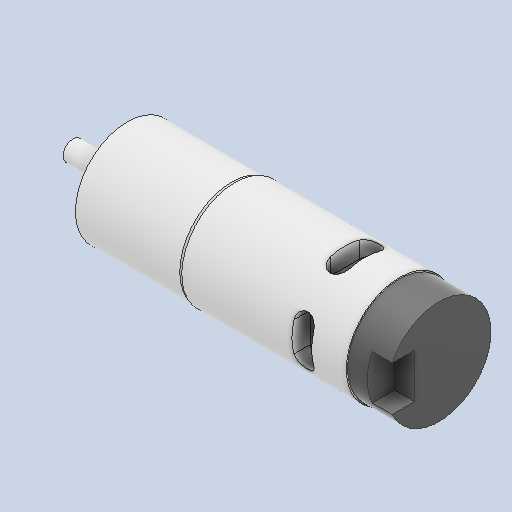
# Autodesk Inventor part: CHP-42GP-775 ABHL
Saved by Autodesk Inventor 2025 (Build 290162000, 162)
## iProperties
Created: 2025-02-16
Part Number: CHP-42GP-775 ABHL
Material: Типовые
Document SubType Name: Modeling
Designer: volko
Density: 1 g/cm^3
Appearance: По умолчанию
Finish1_Area: 8378,395 мм^2
Finish1_Appearance: Smooth - White
Finish2_Area: 1962,332 мм^2
Finish2_Appearance: Glossy - Black
Finish3_Area: 3635,353 мм^2
Finish3_Appearance: Smooth - Black
Finish4_Area: 9380,563 мм^2
Finish4_Appearance: Smooth - White
Author: volko
Autodesk Inventor part; units mm, degrees
ref_plane "YZ Plane" through (0, 0, 0) normal (1, 0, 0) x (0, 1, 0)
ref_plane "XZ Plane" through (0, 0, 0) normal (0, 1, 0) x (-1, 0, 0)
sketch "Эскиз1" plane through (0, 0, 0) normal (0, 0, 1) x (1, 0, 0)
  line L0 (0, 0) -> (0, 4)
  line L1 (0, 4) -> (20, 4)
  line L2 (20, 4) -> (20, 13)
  line L3 (20, 13) -> (22, 13)
  line L4 (22, 13) -> (22, 21)
  line L5 (22, 21) -> (65.5, 21)
  line L6 (65.5, 21.5) -> (132, 21.5)
  line L7 (132, 21.5) -> (132, 21)
  line L8 (132, 21) -> (148, 21)
  line L9 (148, 21) -> (148, 0)
  line L10 (0, 0) -> (148, 0)
  line L11 (65.5, 21) -> (65.5, 21.5)
  point P0 (63, 17.5)
  point P1 (63, 17.5)
  dimension "d5" = 22
  dimension "d6" = 2
  dimension "d7" = 8
  dimension "d8" = 26
  dimension "d9" = 42
  dimension "d11" = 43
  dimension "d12" = 43.5
  dimension "d14" = 66.5
  dimension "d15" = 16
  constraints: 24 end point, 7 perpendicular, 3 vertical, 1 coincident, 1 collinear, 1 parallel, 2 other
  measures "d5" distance between parallel lines of L0 L4
  measures "d6" distance between parallel lines of L2 L4
  measures "d7" diameter of L1 L10
  measures "d8" diameter of L3 L10
  measures "d9" diameter of L5 L10
  measures "d11" diameter of L6 L10
  measures "d12" distance of L4.end L5.end
  measures "d14" distance between parallel lines of L7 L11
  measures "d15" distance of L7.end L8.end
revolve "Вращение1" add sketch "Эскиз1" angle 360 about axis through (0, 0, 0) along (1, 0, 0)
fillet "Сопряжение1" radius 2 1 edges at (65.5, -21, 0)
sketch "Эскиз2" plane through (0, 0, 0) normal (0, 1, 0) x (-1, 0, 0)
  line L0 (0, 4) -> (0, -4) projected
  line L1 (0, -3.5) -> (-12, -3.5)
  line L2 (-12, -3.5) -> (-12, -6.5419)
  line L3 (-12, -6.5419) -> (0, -6.5419)
  line L4 (0, -3.1455) -> (0, -6.5419)
  point P0 (0, 0)
  point P1 (0, 0)
  dimension "d20" = 3.5
  dimension "d21" = 12
  constraints: 8 end point, 2 perpendicular, 2 point on line, 1 horizontal, 1 midpoint, 1 vertical
  measures "d20" distance from line of point (0, 0) L1
  measures "d21" distance of L2.end L3.end
extrude "Выдавливание1" cut sketch "Эскиз2" along normal mid plane 10
ref_plane "РабПлоскость1" through (0, 0, 22) normal (0, 0, 1) x (1, 0, 0)
sketch "Эскиз3" plane through (0, 0, 22) normal (0, 0, 1) x (1, 0, 0)
  line L0 (110, 0) -> (110, -6)
  line L1 (118, -6) -> (118, 0)
  arc A0 (110, -6) -> (118, -6) centre (114, -6) ccw
  line L2 (110, 0) -> (118, 0) construction
  line L3 (110, 0) -> (110, 6)
  line L4 (118, 6) -> (118, 0)
  arc A1 (118, 6) -> (110, 6) centre (114, 6) ccw
  point P0 (0, 0)
  dimension "d23" = 12
  dimension "d24" = 8
  dimension "d25" = 110
  constraints: 10 end point, 4 point on circle, 3 symmetric about line, 3 vertical, 2 centre point, 2 tangent, 1 point on line, 1 other
  measures "d23" distance of A0.centre A1.centre
  measures "d24" distance of L1.end L0.start
  measures "d25" distance of L0.start point (0, 0)
extrude "Выдавливание2" cut sketch "Эскиз3" against normal blind 8
pattern_circular "Круговой массив1" count 4 over 360 about axis through (98.75, 0, 0) along (1, 0, 0) of "Выдавливание2"
sketch "Эскиз4" plane through (0, 0, 22) normal (0, 0, 1) x (1, 0, 0)
  line L0 (148, 9) -> (140, 9)
  line L1 (140, 9) -> (140, -9)
  line L2 (140, -9) -> (148, -9)
  line L3 (148, -21) -> (148, 21) projected
  point P0 (0, 0)
  dimension "d31" = 8
  dimension "d32" = 18
  dimension "d33" = 9
  constraints: 6 end point, 2 perpendicular, 1 horizontal, 1 point on line
  measures "d31" distance between parallel lines of L3 L1
  measures "d32" distance between parallel lines of L0 L2
  measures "d33" distance from line of point (0, 0) L0
extrude "Выдавливание3" cut sketch "Эскиз4" against normal blind 12
sketch "Эскиз5" plane through (22, 0, 0) normal (-1, 0, 0) x (0, 0, 1)
  arc A0 (-3.5, -1.9365) -> (-3.5, 1.9365) centre (0, 0) ccw projected
  circle A1 centre (0, 0) radius 17.5
  line L0 (0, 0) -> (0, -39) construction
  line L1 (0, 0) -> (12.3744, -12.3744) construction
  point P0 (12.3744, 12.3744)
  point P1 (-12.3744, 12.3744)
  point P2 (-12.3744, -12.3744)
  dimension "d43" = 35
  dimension "d44" = 45
  dimension "d47" = 360
  constraints: 4 end point, 1 coincident, 1 vertical, 8 other
  measures "d44" angle of L0 L1
hole "Отверстие1" at (22, -12.3744, 12.3744) at (22, 12.3744, 12.3744) at (22, 12.3744, -12.3744) at (22, -12.3744, -12.3744) direction (1, 0, 0) diameter 3.242 depth 5.2 tip angle 118 thread size "M4x0.7" class "6H" standard "ISO Metric profile"
